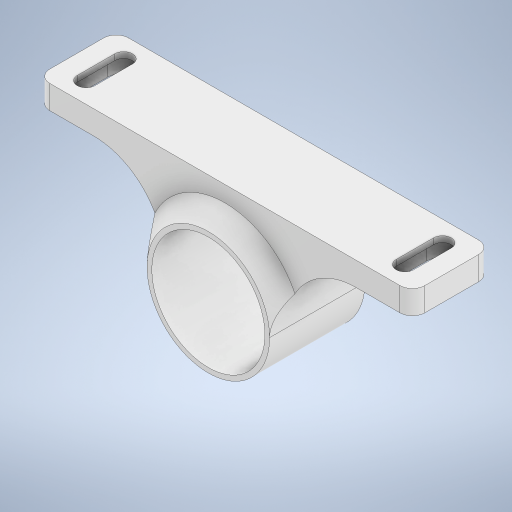
# Autodesk Inventor part: Pillow RevB
Saved by Autodesk Inventor 2024.1 (Build 281209000, 209)
## iProperties
Created: 2023-11-02
Part Number: Pillow RevB
Material: PC/ABS Plastic
Document SubType Name: Modeling
Designer: czb556
Density: 1.1 g/cm^3
Appearance: Smooth - White
Author: czb556
## iProperties of the stored document pillow2_3DPrint.ipt
Created: 2023-11-02
Part Number: pillow2_3DPrint
Material: Generic
Document SubType Name: Modeling
Designer: baloc
Density: 1 g/cm^3
Appearance: Default
Author: baloc
Autodesk Inventor part; units mm, degrees
ref_plane "YZ Plane" through (0, 0, 0) normal (1, 0, 0) x (0, 1, 0)
ref_plane "XZ Plane" through (0, 0, 0) normal (0, 1, 0) x (-1, 0, 0)
ref_plane "XY Plane" through (0, 0, 0) normal (0, 0, 1) x (1, 0, 0)
sketch "Sketch1" plane through (0, 0, 0) normal (0, 0, 1) x (1, 0, 0)
  circle A0 centre (0, 0) radius 15.5575
  line L0 (-47.625, 23.802) -> (47.625, 23.802)
  line L1 (-47.625, 23.802) -> (-47.625, 17.802)
  line L2 (-47.625, 17.802) -> (-33.3595, 17.802)
  line L3 (47.625, 23.802) -> (47.625, 17.802)
  line L4 (47.625, 17.802) -> (33.3595, 17.802)
  arc A1 (33.3595, 17.802) -> (15.5575, 0) centre (33.3595, 0) ccw
  arc A2 (-15.5575, 0) -> (-33.3595, 17.802) centre (-33.3595, 0) ccw
  point P0 (0, 23.802)
  dimension "d0" = 31.115
  dimension "d4" = 95.25
  dimension "d5" = 6
  dimension "d6" = 23.802
  constraints: 10 end point, 6 point on circle, 3 centre point, 2 equal length, 2 horizontal, 2 horizontal alignment, 2 tangent, 2 vertical, 2 vertical alignment, 1 coincident, 1 equal radius, 1 midpoint, 1 perpendicular
  measures "d0" diameter of A0
  measures "d4" distance of L0.start L0.end
  measures "d5" distance of L0.end L3.end
  measures "d6" distance from line of L0 point (0, 0)
extrude "Base" add sketch "Sketch1" along normal mid plane 20
sketch "Sketch2" plane through (0, 0, 10) normal (0, 0, 1) x (1, 0, 0)
  circle A0 centre (0, 0) radius 15.5575
  arc A1 (-15.5575, 0) -> (15.5575, 0) centre (0, 0) ccw projected
  constraints: 1 centre point, 1 coincident, 1 concentric
extrude "Extrusion2" add sketch "Sketch2" along normal blind 4.209
sketch "Sketch7" plane through (0, 0, 14.209) normal (0, 0, 1) x (1, 0, 0)
  circle A0 centre (0, 0) radius 14.351
  dimension "d29" = 28.702
  constraints: 1 centre point, 1 coincident
  measures "d29" diameter of A0
extrude "Bearing hole" cut sketch "Sketch7" against normal blind 25.4
sketch "Sketch3" plane through (-47.625, 17.802, 10) normal (0, -1, 0) x (1, 0, 0)
  line L0 (7.1328, -14.7625) -> (7.1328, -5.2375) construction
  line L1 (9.3828, -14.7625) -> (9.3828, -5.2375)
  line L2 (4.8828, -5.2375) -> (4.8828, -14.7625)
  arc A0 (4.8828, -14.7625) -> (9.3828, -14.7625) centre (7.1328, -14.7625) ccw
  arc A1 (9.3828, -5.2375) -> (4.8828, -5.2375) centre (7.1328, -5.2375) ccw
  line L3 (0, -20) -> (0, 0) projected
  line L4 (14.2655, -20) -> (0, -20) projected
  line L5 (47.625, 14.1524) -> (47.625, -29.8694)
  line L6 (85.8672, -14.7625) -> (85.8672, -5.2375)
  line L7 (90.3673, -5.2375) -> (90.3673, -14.7625)
  arc A2 (85.8672, -14.7625) -> (90.3673, -14.7625) centre (88.1173, -14.7625) ccw
  arc A3 (90.3673, -5.2375) -> (85.8672, -5.2375) centre (88.1173, -5.2375) ccw
  point P0 (47.625, -10)
  point P1 (7.1328, -10)
  point P2 (0, -10)
  point P3 (7.1328, -20)
  dimension "d12" = 4.5
  dimension "d13" = 9.525
  dimension "d20" = 95.25
  constraints: 14 end point, 8 point on circle, 6 symmetric about line, 4 centre point, 4 tangent, 3 midpoint, 2 vertical, 1 horizontal alignment, 1 parallel, 1 vertical alignment, 2 other
  measures "d12" diameter of A1
  measures "d13" distance of L0.start L0.end
  measures "d20" diameter of L3 L5
extrude "Slot" cut sketch "Sketch3" against normal through all
sketch "Sketch4" plane through (-47.625, 17.802, 10) normal (0, -1, 0) x (1, 0, 0)
  line L0 (4.8828, -14.7625) -> (4.8828, -5.2375) projected
  arc A0 (9.3828, -5.2375) -> (4.8828, -5.2375) centre (7.1328, -5.2375) ccw projected
  line L1 (9.3828, -5.2375) -> (9.3828, -14.7625) projected
  arc A1 (4.8828, -14.7625) -> (9.3828, -14.7625) centre (7.1328, -14.7625) ccw projected
  line L2 (14.2655, -20) -> (14.2655, 0) projected
  line L3 (0, 0) -> (14.2655, 0) projected
  line L4 (0, -20) -> (0, 0) projected
  line L5 (14.2655, -20) -> (0, -20) projected
  line L6 (7.1328, -14.7625) -> (7.1328, -5.2375) construction
  line L7 (11.1328, -14.7625) -> (11.1328, -5.2375)
  line L8 (3.1328, -5.2375) -> (3.1328, -14.7625)
  arc A2 (3.1328, -14.7625) -> (11.1328, -14.7625) centre (7.1328, -14.7625) ccw
  arc A3 (11.1328, -5.2375) -> (3.1328, -5.2375) centre (7.1328, -5.2375) ccw
  arc A4 (4.8828, -14.7625) -> (9.3828, -14.7625) centre (7.1328, -14.7625) ccw projected
  line L9 (47.625, 10.1157) -> (47.625, -26.1846)
  line L10 (84.1172, -14.7625) -> (84.1173, -5.2375)
  line L11 (92.1173, -5.2375) -> (92.1173, -14.7625)
  arc A5 (84.1172, -14.7625) -> (92.1173, -14.7625) centre (88.1172, -14.7625) ccw
  arc A6 (92.1173, -5.2375) -> (84.1173, -5.2375) centre (88.1172, -5.2375) ccw
  point P0 (47.625, -10)
  point P1 (7.1328, -10)
  dimension "d17" = 8
  dimension "d21" = 95.25
  constraints: 14 end point, 8 point on circle, 6 symmetric about line, 4 centre point, 4 tangent, 2 parallel, 1 concentric, 1 midpoint, 1 vertical, 2 other
  measures "d17" diameter of A3
  measures "d21" diameter of L4 L9
extrude "Counterbore" cut sketch "Sketch4" against normal blind 4.5 contours L0 A0 L1 A1 | A2 L8 A3 L7 | L10 A6 L11 A5
fillet "Fillet1" radius 3.175 4 edges at (-47.625, 20.802, 10) (-47.625, 20.802, -10) (47.625, 20.802, -10) (47.625, 20.802, 10)
chamfer "Chamfer2" distance 4.209 angle 45 1 edges at (0, 15.5575, 10)
equation "\"d20\" = d4"
equation "\"d21\" = d20"
equation "\"d43\" = d9"
equation "\"d9\" = 4.209"
body "Solid1"
